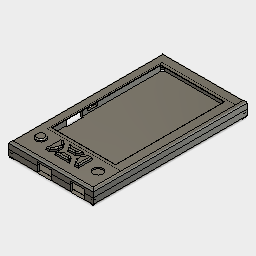
Case_Design (Autodesk Fusion 360 design; units mm, degrees)
Autodesk Fusion 360 part; units mm, degrees
sketch "Screen" plane through (0, 0, 0) normal (0, 1, 0) x (1, 0, 0)
  line L0 (-28.5, 49.35) -> (28.5, 49.35)
  line L1 (28.5, 49.35) -> (28.5, -49.35)
  line L2 (28.5, -49.35) -> (-28.5, -49.35)
  line L3 (-28.5, -49.35) -> (-28.5, 49.35)
  line L4 (-28.5, 49.35) -> (28.5, -49.35) construction
  line L5 (28.5, 49.35) -> (-28.5, -49.35) construction
  line L6 (-31.11, 52.75) -> (36.09, 52.75)
  line L7 (36.09, 52.75) -> (36.09, -52.75)
  line L8 (36.09, -52.75) -> (-31.11, -52.75)
  line L9 (-31.11, -52.75) -> (-31.11, 52.75)
  line L10 (29.5, 50.35) -> (-29.5, 50.35)
  line L11 (-29.5, 50.35) -> (-29.5, -50.35)
  line L12 (-29.5, -50.35) -> (29.5, -50.35)
  line L13 (29.5, -50.35) -> (29.5, 50.35)
  line L14 (29.5, 50.35) -> (-29.5, -50.35) construction
  line L15 (-29.5, 50.35) -> (29.5, -50.35) construction
  dimension "d1" = 98.7
  dimension "d2" = 57
  dimension "d3" = 31.11
  dimension "d4" = 36.09
  dimension "d5" = 52.75
  dimension "d6" = 52.75
  dimension "d14" = 100.7
  dimension "d15" = 59
  measures "d1" distance of L0.end L1.end
  measures "d2" distance of L1.end L2.end
  measures "d3" distance of origin L9
  measures "d4" distance of origin L7
  measures "d5" distance of origin L6
  measures "d6" distance of origin L8
  measures "d14" distance of L10.end L11.end
  measures "d15" distance of L11.end L12.end
extrude "Extrude1" add sketch "Screen" along normal blind 4.4 contours L6 L7 L8 L9 | L10 L11 L12 L13 picked at (33.893333, 16.783333) picked at (-29.166667, -16.45) makes body 1
extrude "Extrude2" add sketch "Screen" along normal blind 4.4 separate body contours L0 L1 L2 L3 picked at (-9.5, 16.45) makes body 2
extrude "Extrude3" add sketch "Screen" along normal blind 2 contours L0 L1 L2 L3 picked at (-9.5, 16.45) bodies 1
move_face "OffsetFaces1" offset -2 1 faces at (-9.5, 0, -16.45) on bodies 2
sketch "Board" plane through (0, 0, 0) normal (0, 1, 0) x (1, 0, 0)
  line L0 (-35.792, 11.9058) -> (36.09, 11.9058)
  line L1 (36.09, 11.9058) -> (36.09, -77.15)
  line L2 (36.09, -77.15) -> (-35.792, -77.15)
  line L3 (-35.792, -77.15) -> (-35.792, 11.9058)
  circle A0 centre (0.149, -59.1922) radius 2.25
  circle A1 centre (0.149, -68.0822) radius 2.25
  circle A2 centre (11.579, -63.6372) radius 2.25
  circle A3 centre (-11.281, -63.6372) radius 2.25
  circle A4 centre (-26.267, -63.6372) radius 2.25
  circle A5 centre (26.565, -63.6372) radius 2.25
  circle A6 centre (-31.651, -73.0942) radius 2
  circle A7 centre (31.949, -73.0942) radius 2
  line L4 (-35.792, -9.58404) -> (-32.192, -9.58404)
  line L5 (-32.192, -9.58404) -> (-32.192, -1.08404)
  line L6 (-32.192, -1.08404) -> (-35.792, -1.08404)
  line L7 (-35.792, -1.08404) -> (-35.792, -9.58404)
  line L8 (-35.792, -9.58404) -> (-32.192, -1.08404) construction
  line L9 (-32.192, -9.58404) -> (-35.792, -1.08404) construction
  line L10 (-35.792, -27.76274) -> (-23.292, -27.76274)
  line L11 (-23.292, -27.76274) -> (-23.292, -16.76274)
  line L12 (-23.292, -16.76274) -> (-35.792, -16.76274)
  line L13 (-35.792, -16.76274) -> (-35.792, -27.76274)
  line L14 (-35.792, -27.76274) -> (-23.292, -16.76274) construction
  line L15 (-23.292, -27.76274) -> (-35.792, -16.76274) construction
  line L16 (28.029, -77.15) -> (20.529, -77.15)
  line L17 (20.529, -77.15) -> (20.529, -71.4)
  line L18 (20.529, -71.4) -> (28.029, -71.4)
  line L19 (28.029, -71.4) -> (28.029, -77.15)
  line L20 (28.029, -77.15) -> (20.529, -71.4) construction
  line L21 (20.529, -77.15) -> (28.029, -71.4) construction
  line L22 (-2.451, -77.15) -> (-9.951, -77.15)
  line L23 (-9.951, -77.15) -> (-9.951, -71.4)
  line L24 (-9.951, -71.4) -> (-2.451, -71.4)
  line L25 (-2.451, -71.4) -> (-2.451, -77.15)
  line L26 (-2.451, -77.15) -> (-9.951, -71.4) construction
  line L27 (-9.951, -77.15) -> (-2.451, -71.4) construction
  line L28 (36.09, -52.75) -> (-31.11, -52.75)
  line L29 (-37.692, -1.441077) -> (-32.192, -1.441077)
  line L30 (-32.192, -1.441077) -> (-32.192, -3.441077)
  line L31 (-32.192, -3.441077) -> (-37.692, -3.441077)
  line L32 (-37.692, -3.441077) -> (-37.692, -1.441077)
  line L33 (-38.692, -17.26274) -> (-23.292, -17.26274)
  line L34 (-23.292, -17.26274) -> (-23.292, -27.26274)
  line L35 (-23.292, -27.26274) -> (-38.692, -27.26274)
  line L36 (-38.692, -27.26274) -> (-38.692, -17.26274)
  line L37 (-35.792, -77.15) -> (36.09, -77.15)
  line L38 (36.09, -77.15) -> (36.09, -40.95)
  line L39 (36.09, -40.95) -> (-35.792, -40.95)
  line L40 (-35.792, -40.95) -> (-35.792, -77.15)
  line L41 (-35.792, -1.08404) -> (-42.092, -1.08404)
  line L42 (-42.092, -1.08404) -> (-42.092, -9.58404)
  line L43 (-42.092, -9.58404) -> (-35.792, -9.58404)
  line L44 (-35.792, -9.58404) -> (-35.792, -1.08404)
  line L45 (-35.792, -27.76274) -> (-35.792, -16.76274)
  line L46 (-9.951, -77.15) -> (-2.451, -77.15)
  line L47 (20.529, -77.15) -> (28.029, -77.15)
  line L48 (-35.792, -14.76274) -> (-42.092, -14.76274)
  line L49 (-42.092, -14.76274) -> (-42.092, -29.76274)
  line L50 (-42.092, -29.76274) -> (-35.792, -29.76274)
  line L51 (-35.792, -29.76274) -> (-35.792, -14.76274)
  line L52 (-12.701, -77.15) -> (0.299, -77.15)
  line L53 (0.299, -77.15) -> (0.299, -83.45)
  line L54 (0.299, -83.45) -> (-12.701, -83.45)
  line L55 (-12.701, -83.45) -> (-12.701, -77.15)
  line L56 (17.779, -77.15) -> (30.779, -77.15)
  line L57 (30.779, -77.15) -> (30.779, -83.45)
  line L58 (30.779, -83.45) -> (17.779, -83.45)
  line L59 (17.779, -83.45) -> (17.779, -77.15)
  point P0 (-33.992, -5.33404)
  point P1 (-29.542, -22.26274)
  point P2 (24.279, -74.275)
  point P3 (-6.201, -74.275)
  dimension "d16" = 71.882
  dimension "d17" = 89.0558
  dimension "d18" = 4.5
  dimension "d19" = 17.9578
  dimension "d20" = 35.941
  dimension "d21" = 4.5
  dimension "d22" = 35.941
  dimension "d23" = 9.0678
  dimension "d24" = 4.5
  dimension "d25" = 13.5128
  dimension "d26" = 4.5
  dimension "d27" = 13.5128
  dimension "d28" = 4.5
  dimension "d29" = 13.5128
  dimension "d30" = 4.5
  dimension "d31" = 13.5128
  dimension "d32" = 11.43
  dimension "d33" = 11.43
  dimension "d34" = 26.416
  dimension "d35" = 26.416
  dimension "d36" = 4
  dimension "d37" = 4.141
  dimension "d38" = 4.0558
  dimension "d39" = 4
  dimension "d40" = 4.141
  dimension "d41" = 4.0558
  dimension "d42" = 17.23984
  dimension "d43" = 12.5
  dimension "d44" = 34.16854
  dimension "d45" = 7.5
  dimension "d46" = 5.75
  dimension "d47" = 11.811
  dimension "d48" = 5.75
  dimension "d49" = 7.5
  dimension "d50" = 5.75
  dimension "d51" = 5.75
  dimension "d52" = 42.291
  dimension "d53" = 36.09
  dimension "d54" = 24.4
  dimension "d57" = 11
  dimension "d58" = 8.5
  dimension "d59" = 3.6
  dimension "d60" = 5.5
  dimension "d61" = 2
  dimension "d62" = 5.5
  dimension "d63" = 15.4
  dimension "d64" = 10
  dimension "d65" = 15.4
  dimension "d66" = 0.5
  dimension "d80" = 36.2
  dimension "d129" = 6.3
  dimension "d161" = 6.3
  dimension "d162" = 15
  dimension "d164" = 2
  dimension "d177" = 13
  dimension "d178" = 6.3
  dimension "d179" = 13
  dimension "d180" = 6.3
  dimension "d181" = 2.75
  dimension "d182" = 2.75
  measures "d16" distance of L0.start L0.end
  measures "d17" distance of L0.start L2.end
  measures "d18" diameter of A0
  measures "d19" distance of L2 A0.centre
  measures "d20" distance of L1 A0.centre
  measures "d21" diameter of A1
  measures "d22" distance of L1 A1.centre
  measures "d23" distance of L2 A1.centre
  measures "d24" diameter of A2
  measures "d25" distance of L2 A2.centre
  measures "d26" diameter of A3
  measures "d27" distance of L2 A3.centre
  measures "d28" diameter of A4
  measures "d29" distance of L2 A4.centre
  measures "d30" diameter of A5
  measures "d31" distance of L2 A5.centre
  measures "d32" distance of A1.centre A3.centre
  measures "d33" distance of A1.centre A2.centre
  measures "d34" distance of A1.centre A4.centre
  measures "d35" distance of A1.centre A5.centre
  measures "d36" diameter of A6
  measures "d37" distance of L3 A6.centre
  measures "d38" distance of L2 A6.centre
  measures "d39" diameter of A7
  measures "d40" distance of L1 A7.centre
  measures "d41" distance of L2 A7.centre
  measures "d45" distance of L17.end L18.end
  measures "d46" distance of L16.end L17.end
  measures "d47" distance of L1 P2
  measures "d48" distance of L2 L18
  measures "d49" distance of L23.end L24.end
  measures "d50" distance of L22.end L23.end
  measures "d51" distance of L2 L24
  measures "d52" distance of L1 P3
  measures "d53" distance of origin L1
  measures "d54" distance of L2 L28
  measures "d57" distance of L10 L12
  measures "d58" distance of L4 L6
  measures "d59" distance of L3 L5
  measures "d62" distance of L5 L32
  measures "d65" distance of L11 L36
  measures "d66" distance of L12 L33
  measures "d80" distance of L2.end L39.end
  measures "d164" distance of L10 L50
  measures "d177" distance of L52.start L52.end
  measures "d178" distance of L52.start L54.end
  measures "d179" distance of L56.start L56.end
  measures "d180" distance of L56.start L58.end
  measures "d181" distance of L23 L55
  measures "d182" distance of L17 L59
extrude "Extrude4" add sketch "Board" against normal blind 1.65 separate body contours L0 L1 L3 L4 L5 L6 L10 L11 L12 L30 L34 L39 L51 | L3 L5 L6 L7 L29 L44 | L1 L2 L3 L17 L18 L19 L23 L24 L25 L37 L38 L39 L40 L52 L56 | L3 L5 L7 L29 L30 L31 L44 | L3 L4 L5 L7 L31 L44 | L3 L10 L11 L13 L35 L45 L51 | L2 L16 L17 L18 L19 L37 L47 L56 | L2 L22 L23 L24 L25 L37 L46 L52 | L3 L11 L13 L33 L34 L35 L45 L51 | L3 L11 L12 L13 L33 L45 L51 | A0 | A1 | A2 | A3 | A4 | A5 picked at (16.296, -15.26898) picked at (-33.392, -1.203052) picked at (0.092952, -46.28283) picked at (-33.392, -2.107744) picked at (-34.592, -7.536386) picked at (-27.458667, -27.596073) picked at (25.529, -73.316667) picked at (-4.951, -75.233333) picked at (-31.625333, -20.596073) picked at (-27.458667, -16.929407) picked at (0.092952, -58.767356) picked at (-0.017891, -67.351004) picked at (11.745891, -64.302315) picked at (-12.078671, -64.273321) picked at (-26.323048, -64.385103) picked at (26.621048, -64.351689) makes body 3
extrude "Extrude5" add sketch "Board" against normal blind 5.25 contours L3 L5 L6 L7 L29 L44 | L3 L5 L7 L29 L30 L31 L44 | L3 L7 L29 L31 L32 L44 | L3 L4 L5 L7 L31 L44 picked at (-33.392, -1.203052) picked at (-33.392, -2.107744) picked at (-37.058667, -2.774411) picked at (-34.592, -7.536386) bodies 3
extrude "Extrude6" add sketch "Board" against normal blind 3.1 contours L3 L10 L11 L13 L35 L45 L51 | L3 L13 L33 L35 L36 L45 L51 | L3 L11 L13 L33 L34 L35 L45 L51 | L3 L11 L12 L13 L33 L45 L51 picked at (-27.458667, -27.596073) picked at (-36.758667, -23.929407) picked at (-31.625333, -20.596073) picked at (-27.458667, -16.929407) bodies 3
extrude "Extrude7" cut sketch "Board" against normal blind 1.65 contours L3 L13 L33 L35 L36 L45 L51 picked at (-36.758667, -23.929407) bodies 3
extrude "Extrude8" cut sketch "Board" against normal blind 2.8 contours L3 L7 L29 L31 L32 L44 picked at (-37.058667, -2.774411) bodies 3
extrude "Extrude9" cut sketch "Board" along normal blind 0.45 from surface at -5.25 contours L3 L7 L29 L31 L32 L44 picked at (-37.058667, -2.774411) bodies 3
extrude "Extrude10" add sketch "Board" against normal blind 4.35 contours L2 L16 L17 L18 L19 L37 L47 L56 | L2 L22 L23 L24 L25 L37 L46 L52 picked at (25.529, -73.316667) picked at (-4.951, -75.233333) bodies 3
extrude "Extrude11" add sketch "Board" against normal blind 1.07 from surface at -5.15 separate body contours L1 L2 L3 L17 L18 L19 L23 L24 L25 L37 L38 L39 L40 L52 L56 | L2 L16 L17 L18 L19 L37 L47 L56 | L2 L22 L23 L24 L25 L37 L46 L52 | A0 | A1 | A2 | A3 | A4 | A5 | A6 picked at (0.092952, -46.28283) picked at (25.529, -73.316667) picked at (-4.951, -75.233333) picked at (0.092952, -58.767356) picked at (-0.017891, -67.351004) picked at (11.745891, -64.302315) picked at (-12.078671, -64.273321) picked at (-26.323048, -64.385103) picked at (26.621048, -64.351689) picked at (-31.140127, -73.843513) makes body 4
move_face "OffsetFaces2" offset 4 1 faces at (33.909345, -5.863333, 73.490492) on bodies 4
sketch "Case" plane through (0, 0, 0) normal (0, 1, 0) x (1, 0, 0)
  line L0 (-36.792, 59.65) -> (37.09, 59.65)
  line L1 (37.09, 59.65) -> (37.09, -78.65)
  line L2 (37.09, -78.65) -> (-36.792, -78.65)
  line L3 (-36.792, -78.65) -> (-36.792, 59.65)
  line L4 (36.09, 11.9058) -> (36.09, -77.15)
  line L5 (-35.792, -77.15) -> (36.09, -77.15)
  line L6 (-35.792, -40.95) -> (-35.792, -77.15)
  line L7 (-31.11, 52.75) -> (36.09, 52.75)
  line L8 (-38.792, 61.65) -> (39.09, 61.65)
  line L9 (39.09, 61.65) -> (39.09, -80.65)
  line L10 (39.09, -80.65) -> (-38.792, -80.65)
  line L11 (-38.792, -80.65) -> (-38.792, 61.65)
  circle A0 centre (-31.651, -73.0942) radius 1.35
  circle A1 centre (31.949, -73.0942) radius 1.35
  circle A2 centre (-31.651, -73.0942) radius 3
  circle A3 centre (31.949, -73.0942) radius 3
  circle A4 centre (-36.792, -78.65) radius 0.825
  circle A5 centre (-36.792, -78.65) radius 1.85
  circle A6 centre (37.09, -78.65) radius 0.825
  circle A7 centre (37.09, -78.65) radius 1.85
  circle A8 centre (-36.792, 59.65) radius 0.825
  circle A9 centre (-36.792, 59.65) radius 1.85
  circle A10 centre (37.09, 59.65) radius 0.825
  circle A11 centre (37.09, 59.65) radius 1.85
  line L12 (36.59, -77.65) -> (-36.292, -77.65)
  line L13 (-36.292, -77.65) -> (-36.292, -75.498152)
  line L14 (36.59, -77.65) -> (36.59, -75.817932)
  point P0 (-31.651, -73.0942)
  point P1 (31.949, -73.0942)
  dimension "d85" = 1
  dimension "d86" = 1.5
  dimension "d87" = 1
  dimension "d88" = 6.9
  dimension "d89" = 2
  dimension "d90" = 2
  dimension "d91" = 2
  dimension "d92" = 2
  dimension "d102" = 2.7
  dimension "d103" = 2.7
  dimension "d104" = 6
  dimension "d105" = 6
  dimension "d195" = 1.65
  dimension "d196" = 3.7
  dimension "d197" = 1.65
  dimension "d198" = 3.7
  dimension "d199" = 1.65
  dimension "d200" = 3.7
  dimension "d201" = 1.65
  dimension "d202" = 3.7
  dimension "d203" = 0.5
  dimension "d204" = 0.5
  dimension "d205" = 0.5
  measures "d85" distance of L1 L4
  measures "d86" distance of L2 L5
  measures "d87" distance of L3 L6
  measures "d88" distance of L0 L7
  measures "d89" distance of L2 L10
  measures "d90" distance of L1 L9
  measures "d91" distance of L3 L11
  measures "d92" distance of L0 L8
  measures "d102" diameter of A0
  measures "d103" diameter of A1
  measures "d104" diameter of A2
  measures "d105" diameter of A3
  measures "d195" diameter of A4
  measures "d196" diameter of A5
  measures "d197" diameter of A6
  measures "d198" diameter of A7
  measures "d199" diameter of A8
  measures "d200" diameter of A9
  measures "d201" diameter of A10
  measures "d202" diameter of A11
  measures "d203" distance of L6 L13
  measures "d204" distance of L5 L12
  measures "d205" distance of L4 L14
extrude "Extrude12" add sketch "Case" along normal blind 4.85 separate body contours L0 L3 A8 | L0 L3 A8 | L0 L3 A8 A9 | L0 L3 A8 A9 | L0 L1 L3 L5 A5 A7 A9 A11 | L0 L1 A10 A11 | L0 L1 A10 A11 | L2 L3 A4 A5 L12 L13 | L2 L3 A4 A5 | L0 L1 A10 | L0 L1 A10 | L2 L3 A4 | L2 L3 A4 | L5 L6 A5 L12 L13 | L2 A5 A7 L12 | L1 L2 A6 A7 | L1 L2 A6 A7 L12 L14 | L5 L6 A5 | L5 A5 A7 L12 | L1 L2 A6 | L1 L2 A6 | L4 L5 A7 L12 L14 | L4 L5 A7 | L8 L9 L10 L11 | A0 | A1 | A2 | A3 picked at (-37.189257, 59.27178) picked at (-36.244799, 59.610863) picked at (-38.236361, 60.070699) picked at (-35.906098, 58.433837) picked at (10.383659, 15.233899) picked at (35.591626, 59.782896) picked at (36.012293, 58.600037) picked at (-35.898689, -77.803247) picked at (-38.22667, -78.197355) picked at (36.852031, 60.144147) picked at (36.542799, 59.610863) picked at (-36.310506, -78.387085) picked at (-37.340345, -78.636539) picked at (-35.87162, -77.365492) picked at (11.846, -78.474515) picked at (35.588554, -78.741909) picked at (36.196689, -77.803247) picked at (-35.782685, -77.118479) picked at (11.943854, -77.526007) picked at (36.543072, -78.690987) picked at (36.575991, -78.458284) picked at (36.16962, -77.365492) picked at (36.080685, -77.118479) picked at (-37.006166, 12.933333) picked at (-31.751134, -72.655482) picked at (32.065167, -73.161269) picked at (-29.389022, -74.018087) picked at (29.687022, -74.018087) makes body 5
extrude "Extrude13" cut sketch "Screen" along normal blind 5 contours L0 L1 L2 L3 | L10 L11 L12 L13 picked at (-9.5, 16.45) picked at (-29.166667, -16.45) bodies 5
extrude "Extrude14" cut sketch "Screen" along normal blind 4.65 contours L0 L1 L2 L3 | L6 L7 L8 L9 | L10 L11 L12 L13 picked at (-9.5, 16.45) picked at (33.893333, 16.783333) picked at (-29.166667, -16.45) bodies 5
extrude "Extrude15" cut sketch "Case" along normal blind 4 contours L0 L3 A8 | L0 L3 A8 A9 | L0 L1 L3 L5 A5 A7 A9 A11 | L0 L1 A10 A11 | L2 L3 A4 A5 L12 L13 | L0 L1 A10 | L2 L3 A4 | L5 L6 A5 L12 L13 | L2 A5 A7 L12 | L1 L2 A6 A7 L12 L14 | L5 L6 A5 | L5 A5 A7 L12 | L1 L2 A6 | L4 L5 A7 L12 L14 | L4 L5 A7 | A0 | A1 | A2 | A3 picked at (-36.244799, 59.610863) picked at (-35.906098, 58.433837) picked at (10.383659, 15.233899) picked at (36.012293, 58.600037) picked at (-35.898689, -77.803247) picked at (36.542799, 59.610863) picked at (-36.310506, -78.387085) picked at (-35.87162, -77.365492) picked at (11.846, -78.474515) picked at (36.196689, -77.803247) picked at (-35.782685, -77.118479) picked at (11.943854, -77.526007) picked at (36.575991, -78.458284) picked at (36.16962, -77.365492) picked at (36.080685, -77.118479) picked at (-31.751134, -72.655482) picked at (32.065167, -73.161269) picked at (-29.389022, -74.018087) picked at (29.687022, -74.018087) bodies 5
extrude "Extrude16" add sketch "Case" along normal blind 4.45 contours A2 | A3 picked at (-29.389022, -74.018087) picked at (29.687022, -74.018087) bodies 5
move_face "OffsetFaces5" offset -1 1 faces at (36.09, 4.216667, -17.583333) on bodies 5
extrude "Extrude17" add 1 faces at (11.909948, 4, 58.851227) along direction (0, -1, 0) blind 0.2 on bodies 5 bodies 5
extrude "Extrude18" cut 1 faces at (14.356667, 4.366667, -52.75) along direction (0, 0, -1) blind 0.4 on bodies 5 bodies 5
extrude "Extrude19" add 1 faces at (9.932667, 4.85, 70.55) along direction (0, 1, 0) blind 0.2 on bodies 5 bodies 5
extrude "Extrude20" cut 2 faces at (32.029302, 4, 72.742376) (-31.550866, 4, 73.532918) along direction (0, 1, 0) blind 0.2 on bodies 5 bodies 5
extrude "Extrude21" cut 1 faces at (14.356667, 4.366667, -53.15) along direction (0, 0, -1) blind 0.05 on bodies 5 bodies 5
extrude "Extrude22" add 1 faces at (9.932667, 5.05, 70.55) along direction (0, 1, 0) blind 0.1 on bodies 5 bodies 5
extrude "Extrude23" cut 2 faces at (32.029302, 4.2, 72.742376) (-31.550866, 4.2, 73.532918) along direction (0, 1, 0) blind 0.1 on bodies 5 bodies 5
extrude "Extrude24" add sketch "Case" against normal blind 7.3 separate body contours L0 L3 A8 | L0 L3 A8 A9 | L0 L1 A10 A11 | L2 L3 A4 A5 | L0 L1 A10 | L2 L3 A4 | L1 L2 A6 A7 | L1 L2 A6 | L8 L9 L10 L11 picked at (-37.189257, 59.27178) picked at (-38.236361, 60.070699) picked at (35.591626, 59.782896) picked at (-38.22667, -78.197355) picked at (36.852031, 60.144147) picked at (-37.340345, -78.636539) picked at (35.588554, -78.741909) picked at (36.543072, -78.690987) picked at (-37.006166, 12.933333) makes body 6
extrude "Extrude25" add sketch "Case" against normal blind 0.5 from surface at -7.3 contours L0 L3 A8 | L0 L3 A8 | L0 L3 A8 A9 | L0 L3 A8 A9 | L0 L1 L3 L5 A5 A7 A9 A11 | L0 L1 A10 A11 | L0 L1 A10 A11 | L2 L3 A4 A5 L12 L13 | L2 L3 A4 A5 | L0 L1 A10 | L0 L1 A10 | L2 L3 A4 | L2 L3 A4 | L5 L6 A5 L12 L13 | L2 A5 A7 L12 | L1 L2 A6 A7 | L1 L2 A6 A7 L12 L14 | L5 L6 A5 | L5 A5 A7 L12 | L1 L2 A6 | L1 L2 A6 | L4 L5 A7 L12 L14 | L4 L5 A7 | L8 L9 L10 L11 | A0 | A1 | A2 | A3 picked at (-37.189257, 59.27178) picked at (-36.244799, 59.610863) picked at (-38.236361, 60.070699) picked at (-35.906098, 58.433837) picked at (10.383659, 15.233899) picked at (35.591626, 59.782896) picked at (36.012293, 58.600037) picked at (-35.898689, -77.803247) picked at (-38.22667, -78.197355) picked at (36.852031, 60.144147) picked at (36.542799, 59.610863) picked at (-36.310506, -78.387085) picked at (-37.340345, -78.636539) picked at (-35.87162, -77.365492) picked at (11.846, -78.474515) picked at (35.588554, -78.741909) picked at (36.196689, -77.803247) picked at (-35.782685, -77.118479) picked at (11.943854, -77.526007) picked at (36.543072, -78.690987) picked at (36.575991, -78.458284) picked at (36.16962, -77.365492) picked at (36.080685, -77.118479) picked at (-37.006166, 12.933333) picked at (-31.751134, -72.655482) picked at (32.065167, -73.161269) picked at (-29.389022, -74.018087) picked at (29.687022, -74.018087) bodies 6
extrude "Extrude26" cut sketch "Board" against normal blind 3 contours L0 L1 L3 L4 L5 L6 L10 L11 L12 L30 L34 L39 L51 | L3 L5 L6 L7 L29 L44 | L3 L7 L29 L31 L32 L41 L42 L43 L44 | L1 L2 L3 L17 L18 L19 L23 L24 L25 L37 L38 L39 L40 L52 L56 | L3 L5 L7 L29 L30 L31 L44 | L3 L7 L29 L31 L32 L44 | L3 L4 L5 L7 L31 L44 | L3 L10 L11 L13 L35 L45 L51 | L2 L16 L17 L18 L19 L37 L47 L56 | L2 L22 L23 L24 L25 L37 L46 L52 | L3 L11 L13 L33 L34 L35 L45 L51 | L3 L11 L12 L13 L33 L45 L51 | A0 | A1 | A2 | A3 | A4 | A5 | A6 | A7 picked at (16.296, -15.26898) picked at (-33.392, -1.203052) picked at (-38.525333, -7.536386) picked at (0.092952, -46.28283) picked at (-33.392, -2.107744) picked at (-37.058667, -2.774411) picked at (-34.592, -7.536386) picked at (-27.458667, -27.596073) picked at (25.529, -73.316667) picked at (-4.951, -75.233333) picked at (-31.625333, -20.596073) picked at (-27.458667, -16.929407) picked at (0.092952, -58.767356) picked at (-0.017891, -67.351004) picked at (11.745891, -64.302315) picked at (-12.078671, -64.273321) picked at (-26.323048, -64.385103) picked at (26.621048, -64.351689) picked at (-31.140127, -73.843513) picked at (32.579264, -73.579959) bodies 6
extrude "Extrude27" cut 2 faces at (-38.125333, -3, 3.917373) (-38.125333, -3, 3.917373) along direction (0, -1, 0) blind 2 on bodies 6 bodies 6
extrude "Extrude28" cut sketch "Board" against normal blind 3 contours L1 L2 L3 L17 L18 L19 L23 L24 L25 L37 L38 L39 L40 L52 L56 | L2 L16 L17 L18 L19 L37 L47 L56 | L2 L22 L23 L24 L25 L37 L46 L52 | A0 | A1 | A2 | A3 | A4 | A5 | A6 | A7 picked at (0.092952, -46.28283) picked at (25.529, -73.316667) picked at (-4.951, -75.233333) picked at (0.092952, -58.767356) picked at (-0.017891, -67.351004) picked at (11.745891, -64.302315) picked at (-12.078671, -64.273321) picked at (-26.323048, -64.385103) picked at (26.621048, -64.351689) picked at (-31.140127, -73.843513) picked at (32.579264, -73.579959) bodies 6
sketch "Buttons" plane through (0, 0, 0) normal (0, 1, 0) x (1, 0, 0)
  line L0 (3.649, -56.6922) -> (-3.351, -56.6922)
  line L1 (-3.351, -56.6922) -> (-3.351, -61.6922) construction
  line L2 (-3.351, -61.6922) -> (3.649, -61.6922)
  line L3 (3.649, -61.6922) -> (3.649, -56.6922) construction
  line L4 (3.649, -56.6922) -> (-3.351, -61.6922) construction
  line L5 (-3.351, -56.6922) -> (3.649, -61.6922) construction
  line L6 (3.649, -65.5822) -> (-3.351, -65.5822)
  line L7 (-3.351, -65.5822) -> (-3.351, -70.5822) construction
  line L8 (-3.351, -70.5822) -> (3.649, -70.5822)
  line L9 (3.649, -70.5822) -> (3.649, -65.5822) construction
  line L10 (3.649, -65.5822) -> (-3.351, -70.5822) construction
  line L11 (-3.351, -65.5822) -> (3.649, -70.5822) construction
  line L12 (3.649, -70.5822) -> (7.149, -70.5822)
  line L13 (-3.351, -70.5822) -> (-6.851, -70.5822)
  line L14 (-6.851, -70.5822) -> (-3.351, -65.5822)
  line L15 (7.149, -70.5822) -> (3.649, -65.5822)
  line L16 (3.649, -56.6922) -> (7.149, -56.6922)
  line L17 (-3.351, -56.6922) -> (-6.851, -56.6922)
  line L18 (-6.851, -56.6922) -> (-3.351, -61.6922)
  line L19 (7.149, -56.6922) -> (3.649, -61.6922)
  line L20 (15.079, -61.6872) -> (8.079, -61.6872) construction
  line L21 (8.079, -61.6872) -> (8.079, -65.5872)
  line L22 (8.079, -65.5872) -> (15.079, -65.5872) construction
  line L23 (15.079, -65.5872) -> (15.079, -61.6872)
  line L24 (15.079, -61.6872) -> (8.079, -65.5872) construction
  line L25 (8.079, -61.6872) -> (15.079, -65.5872) construction
  line L26 (8.079, -65.5872) -> (11.519774, -70.502592)
  line L27 (11.519774, -70.502592) -> (15.079, -70.502592)
  line L28 (8.079, -61.6872) -> (11.519774, -56.771808)
  line L29 (11.519774, -56.771808) -> (15.079, -56.771808)
  line L30 (15.079, -56.771808) -> (15.079, -61.6872)
  line L31 (15.079, -70.502592) -> (15.079, -65.5872)
  line L32 (-7.781, -61.6872) -> (-14.781, -61.6872) construction
  line L33 (-14.781, -61.6872) -> (-14.781, -65.5872)
  line L34 (-14.781, -65.5872) -> (-7.781, -65.5872) construction
  line L35 (-7.781, -65.5872) -> (-7.781, -61.6872)
  line L36 (-7.781, -61.6872) -> (-14.781, -65.5872) construction
  line L37 (-14.781, -61.6872) -> (-7.781, -65.5872) construction
  line L38 (-7.781, -61.6872) -> (-11.221774, -56.771808)
  line L39 (-11.221774, -56.771808) -> (-14.781, -56.771808)
  line L40 (-14.781, -56.771808) -> (-14.781, -61.6872)
  line L41 (-7.781, -65.5872) -> (-11.221774, -70.502592)
  line L42 (-11.221774, -70.502592) -> (-14.781, -70.502592)
  line L43 (-14.781, -70.502592) -> (-14.781, -65.5872)
  circle A0 centre (26.565, -63.6372) radius 4.5
  circle A1 centre (-26.267, -63.6372) radius 4.5
  circle A2 centre (-26.267, -63.6372) radius 4.3
  circle A3 centre (-26.267, -63.6372) radius 1.25
  circle A4 centre (-11.281, -63.6372) radius 1.25
  circle A5 centre (0.149, -59.1922) radius 1.25
  circle A6 centre (0.149, -68.0822) radius 1.25
  circle A7 centre (11.579, -63.6372) radius 1.25
  circle A8 centre (26.565, -63.6372) radius 4.3
  circle A9 centre (26.565, -63.6372) radius 1.25
  line L44 (-17.781, -53.6922) -> (18.079, -53.6922)
  line L45 (18.079, -53.6922) -> (18.079, -73.5822)
  line L46 (18.079, -73.5822) -> (-17.781, -73.5822)
  line L47 (-17.781, -73.5822) -> (-17.781, -53.6922)
  circle A10 centre (-26.267, -63.6372) radius 6.25
  line L48 (-5.759867, -57.0922) -> (5.562729, -57.0922)
  line L49 (-2.287861, -61.2922) -> (1.357745, -61.2922)
  line L50 (6.629845, -56.736333) -> (3.823255, -60.745747)
  line L51 (-6.297632, -56.785208) -> (-3.276985, -61.100418)
  line L52 (-2.287861, -61.2922) -> (-3.425784, -61.2922)
  line L53 (-3.276985, -61.100418) -> (-3.142738, -61.2922)
  line L54 (-5.759867, -57.0922) -> (-6.54032, -57.0922)
  line L55 (-6.297632, -56.785208) -> (-6.303023, -56.777508)
  line L56 (5.562729, -57.0922) -> (6.380738, -57.0922)
  line L57 (3.823255, -60.745747) -> (3.3493, -61.422826)
  line L58 (1.357745, -61.2922) -> (3.440738, -61.2922)
  line L59 (8.479, -62.046318) -> (8.479, -65.111551)
  line L60 (8.740137, -65.834164) -> (11.725664, -70.099203)
  line L61 (12.282208, -70.102592) -> (14.522186, -70.102592)
  line L62 (14.679, -69.606243) -> (14.679, -57.595836)
  line L63 (14.536922, -57.171808) -> (12.223261, -57.171808)
  line L64 (11.623844, -57.320655) -> (8.695281, -61.504316)
  line L65 (14.679, -57.595836) -> (14.679, -56.836265)
  line L66 (11.623844, -57.320655) -> (11.970044, -56.826083)
  line L67 (8.695281, -61.504316) -> (8.202168, -62.208763)
  line L68 (8.740137, -65.834164) -> (8.205868, -65.070923)
  line L69 (8.479, -65.111551) -> (8.479, -65.461111)
  line L70 (12.282208, -70.102592) -> (11.477234, -70.102592)
  line L71 (11.725664, -70.099203) -> (11.728036, -70.102592)
  line L72 (14.679, -69.606243) -> (14.679, -70.426864)
  line L73 (14.522186, -70.102592) -> (14.679, -70.102592)
  line L74 (14.536922, -57.171808) -> (14.679, -57.171808)
  line L75 (12.223261, -57.171808) -> (11.728036, -57.171808)
  line L76 (-6.405298, -70.643) -> (-3.068324, -65.875894)
  line L77 (-2.80703, -65.9822) -> (3.520319, -65.9822)
  line L78 (3.628301, -66.250147) -> (6.683218, -70.614314)
  line L79 (6.421738, -70.1822) -> (-5.596015, -70.1822)
  line L80 (-5.596015, -70.1822) -> (-6.082738, -70.1822)
  line L81 (-2.80703, -65.9822) -> (-3.142738, -65.9822)
  line L82 (3.520319, -65.9822) -> (3.713792, -65.9822)
  line L83 (3.628301, -66.250147) -> (3.440738, -65.9822)
  line L84 (6.421738, -70.1822) -> (6.380738, -70.1822)
  line L85 (-14.381, -56.925456) -> (-14.381, -70.342445)
  line L86 (-14.262215, -70.102592) -> (-11.314217, -70.102592)
  line L87 (-11.291819, -69.905138) -> (-8.288132, -65.614157)
  line L88 (-8.181, -62.073669) -> (-8.181, -65.194233)
  line L89 (-8.293888, -61.652021) -> (-11.525249, -57.03579)
  line L90 (-11.515543, -57.171808) -> (-14.391639, -57.171808)
  line L91 (-14.391639, -57.171808) -> (-14.381, -57.171808)
  line L92 (-11.515543, -57.171808) -> (-11.430036, -57.171808)
  line L93 (-8.181, -62.073669) -> (-8.181, -61.516626)
  line L94 (-8.293888, -61.652021) -> (-8.181, -61.813289)
  line L95 (-8.181, -65.194233) -> (-8.181, -65.701633)
  line L96 (-8.288132, -65.614157) -> (-8.181, -65.461111)
  line L97 (-11.314217, -70.102592) -> (-11.175918, -70.102592)
  line L98 (-11.291819, -69.905138) -> (-11.430036, -70.102592)
  line L99 (-14.262215, -70.102592) -> (-14.381, -70.102592)
  line L100 (8.479, -62.046318) -> (8.479, -61.813289)
  point P0 (0.149, -59.1922)
  point P1 (0.149, -59.1922)
  point P2 (0.149, -68.0822)
  point P3 (0.149, -68.0822)
  point P4 (11.579, -63.6372)
  point P5 (11.579, -63.6372)
  point P6 (-11.281, -63.6372)
  point P7 (-11.281, -63.6372)
  point P8 (26.565, -63.6372)
  point P9 (-26.267, -63.6372)
  dimension "d143" = 5
  dimension "d144" = 7
  dimension "d145" = 5
  dimension "d146" = 7
  dimension "d147" = 3.5
  dimension "d148" = 3.5
  dimension "d149" = 3.5
  dimension "d150" = 3.5
  dimension "d151" = 3.9
  dimension "d152" = 7
  dimension "d153" = 6
  dimension "d154" = 6
  dimension "d155" = 7
  dimension "d156" = 3.9
  dimension "d157" = 6
  dimension "d158" = 6
  dimension "d159" = 9
  dimension "d160" = 9
  dimension "d252" = 8.6
  dimension "d256" = 2.5
  dimension "d257" = 2.5
  dimension "d258" = 2.5
  dimension "d259" = 2.5
  dimension "d260" = 2.5
  dimension "d261" = 8.6
  dimension "d262" = 2.5
  dimension "d263" = 3
  dimension "d264" = 3
  dimension "d265" = 3
  dimension "d266" = 3
  dimension "d267" = 12.5
  dimension "d278" = 0.4
  dimension "d279" = 0.4
  dimension "d280" = 0.4
  dimension "d281" = 0.4
  dimension "d282" = 0.4
  dimension "d283" = 0.4
  dimension "d284" = 0.4
  dimension "d285" = 0.4
  dimension "d286" = 0.4
  dimension "d287" = 0.4
  dimension "d288" = 0.4
  dimension "d289" = 0.4
  dimension "d290" = 0.4
  dimension "d291" = 0.4
  dimension "d292" = 0.4
  dimension "d293" = 0.4
  dimension "d294" = 0.4
  dimension "d295" = 0.4
  dimension "d296" = 0.4
  dimension "d297" = 0.4
  measures "d143" distance of L0.end L1.end
  measures "d144" distance of L1.end L2.end
  measures "d145" distance of L6.end L7.end
  measures "d146" distance of L7.end L8.end
  measures "d147" distance of L8.end L12.end
  measures "d148" distance of L7.end L13.end
  measures "d149" distance of L0.start L16.end
  measures "d150" distance of L0.end L17.end
  measures "d151" distance of L20.end L21.end
  measures "d152" distance of L21.end L22.end
  measures "d155" distance of L33.end L34.end
  measures "d156" distance of L32.end L33.end
  measures "d159" diameter of A0
  measures "d160" diameter of A1
  measures "d252" diameter of A2
  measures "d256" diameter of A3
  measures "d257" diameter of A4
  measures "d258" diameter of A5
  measures "d259" diameter of A6
  measures "d260" diameter of A7
  measures "d261" diameter of A8
  measures "d262" diameter of A9
  measures "d263" distance of L0 L44
  measures "d264" distance of L8 L46
  measures "d265" distance of L23 L45
  measures "d266" distance of L33 L47
  measures "d267" diameter of A10
  measures "d278" distance of L0 L48
  measures "d279" distance of L2 L49
  measures "d280" distance of L19 L50
  measures "d281" distance of L18 L51
  measures "d282" distance of L28 L64
  measures "d283" distance of L29 L63
  measures "d284" distance of L30 L62
  measures "d285" distance of L27 L61
  measures "d286" distance of L26 L60
  measures "d287" distance of L21 L59
  measures "d288" distance of L14 L76
  measures "d289" distance of L6 L77
  measures "d290" distance of L15 L78
  measures "d291" distance of L13 L79
  measures "d292" distance of L43 L85
  measures "d293" distance of L42 L86
  measures "d294" distance of L41 L87
  measures "d295" distance of L35 L88
  measures "d296" distance of L38 L89
  measures "d297" distance of L39 L90
extrude "Extrude30" cut sketch "Buttons" along normal blind 6 contours L0 L2 L16 L17 L18 L19 | L6 L12 L13 L14 L15 L76 L77 L78 L81 L83 | L8 L12 L13 L76 L78 L79 L80 | L76 L77 L78 L79 L80 L81 L83 | L21 L23 L26 L27 L28 L29 L30 L31 | L33 L35 L38 L39 L40 L41 L42 L43 | A0 | A1 | A2 | A3 | A4 | A5 | A6 | A7 | A8 | A9 | L48 L49 L50 L51 L52 L53 L54 L56 L57 L58 | L59 L60 L61 L62 L63 L64 L65 L66 L67 L68 L69 L70 L71 L72 L73 L74 L75 L100 | L85 L86 L87 L88 L89 L90 L92 L93 L94 L95 L96 L98 L99 picked at (-1.182713, -56.958867) picked at (5.726246, -68.7822) picked at (-0.855426, -70.315533) picked at (-3.275264, -68.144301) picked at (14.812333, -64.263093) picked at (-14.514333, -62.9872) picked at (25.36426, -67.893299) picked at (-23.338519, -66.950831) picked at (-23.00433, -63.912928) picked at (-26.007213, -63.78087) picked at (-11.373717, -63.321732) picked at (-0.516997, -59.502625) picked at (0.117862, -68.967135) picked at (11.838787, -63.78087) picked at (29.82767, -63.912928) picked at (26.824787, -63.78087) picked at (-3.37463, -59.066172) picked at (10.588883, -66.929742) picked at (-12.43057, -68.269507) bodies 5
extrude "Extrude31" add 1 faces at (38.423333, 0, 32.55) along direction (0, -1, 0) blind 1.67 on bodies 5 bodies 5
extrude "Extrude32" cut sketch "Board" along normal blind 0.5 from surface at -1.67 contours L3 L13 L33 L35 L36 L45 L48 L49 L50 L51 | L3 L13 L33 L35 L36 L45 L51 picked at (-40.958667, -23.929407) picked at (-36.758667, -23.929407) bodies 5
extrude "Extrude33" cut 3 faces at (38.423333, 0, 32.55) (38.423333, 0, 32.55) (38.423333, 0, 32.55) along direction (0, -1, 0) blind 1.67 on bodies 6 bodies 6
extrude "Extrude34" cut sketch "Board" against normal blind 8 contours L3 L13 L33 L35 L36 L45 L48 L49 L50 L51 | L3 L13 L33 L35 L36 L45 L51 picked at (-40.958667, -23.929407) picked at (-36.758667, -23.929407) bodies 6
fillet "Fillet1" radius 2 5 edges at (0.149, -7.8, -61.65) (39.09, -7.8, 9.5) (0.149, -7.8, 80.65) (-38.792, -7.8, 55.20637) (-38.792, -7.8, -23.44363) on bodies 6
extrude "Extrude35" cut sketch "Board" against normal blind 3 from surface at -4.35 contours L2 L22 L37 L46 L52 L53 L54 L55 picked at (-4.951, -81.35) bodies 6
extrude "Extrude36" cut sketch "Board" against normal blind 3 from surface at -4.35 contours L2 L16 L37 L47 L56 L57 L58 L59 picked at (25.529, -81.35) bodies 6
extrude "Extrude37" cut sketch "Board" along normal blind 3 from surface at -1.65 contours L2 L16 L37 L47 L56 L57 L58 L59 | L2 L22 L37 L46 L52 L53 L54 L55 picked at (25.529, -81.35) picked at (-4.951, -81.35) bodies 5
extrude "Extrude38" cut 2 faces at (-8.367667, -4.35, 79.983333) (22.112333, -4.35, 79.316667) along direction (0, 1, 0) blind 3 on bodies 6 bodies 5 6
fillet "Fillet2" radius 2 4 edges at (-38.792, 5.15, 9.5) (0.149, 5.15, 80.65) (39.09, 5.15, 9.5) (0.149, 5.15, -61.65) on bodies 5
extrude "Extrude39" add sketch "Case" against normal blind 5.5 from surface at 3.8 contours L1 L2 A6 A7 | L1 L2 A6 A7 L12 L14 picked at (35.588554, -78.741909) picked at (36.196689, -77.803247) bodies 5
extrude "Extrude40" cut 1 faces at (36.202931, -1.7, 77.796286) along direction (0, 1, 0) blind 0.03 on bodies 5 bodies 5
extrude "Extrude41" cut sketch "Case" against normal blind 6.6 from surface at 3.8 contours L1 L2 A6 | L1 L2 A6 picked at (36.543072, -78.690987) picked at (36.575991, -78.458284) bodies 5
extrude "Extrude42" add sketch "Case" against normal blind 5.47 from surface at 3.8 contours L2 L3 A4 A5 L12 L13 | L2 L3 A4 A5 picked at (-35.898689, -77.803247) picked at (-38.22667, -78.197355) bodies 5
extrude "Extrude43" cut sketch "Case" against normal blind 7 from surface at 3.8 contours L2 L3 A4 | L2 L3 A4 picked at (-36.310506, -78.387085) picked at (-37.340345, -78.636539) bodies 5
extrude "Extrude44" add sketch "Case" against normal blind 5.47 from surface at 3.8 contours L0 L3 A8 A9 | L0 L3 A8 A9 picked at (-38.236361, 60.070699) picked at (-35.906098, 58.433837) bodies 5
extrude "Extrude45" cut sketch "Case" against normal blind 9 from surface at 3.8 contours L0 L3 A8 | L0 L3 A8 picked at (-37.189257, 59.27178) picked at (-36.244799, 59.610863) bodies 5
extrude "Extrude46" add sketch "Case" against normal blind 5.47 from surface at 3.8 contours L0 L1 A10 A11 | L0 L1 A10 A11 picked at (35.591626, 59.782896) picked at (36.012293, 58.600037) bodies 5
extrude "Extrude47" cut sketch "Case" against normal blind 8.2 from surface at 3.8 contours L0 L1 A10 | L0 L1 A10 picked at (36.852031, 60.144147) picked at (36.542799, 59.610863) bodies 5
delete_face "DeleteFace1" 5 faces at (-37.013976, -7.787643, 62.48071) (-37.013976, -7.787643, -34.972217) (12.462667, -7.783833, 78.903783) (38.437597, -7.277831, 32.922351) (-12.164667, -7.783833, -59.903783) on bodies 6
extrude "Extrude48" add 1 faces at (14.129333, -7.8, 11.254247) along direction (0, -1, 0) blind 1 on bodies 6 bodies 6
fillet "Fillet3" radius 2 5 edges at (-38.792, -8.8, 55.20637) (0.149, -8.8, 80.65) (39.09, -8.8, 9.5) (0.149, -8.8, -61.65) (-38.792, -8.8, -23.44363) on bodies 6
extrude "Extrude49" add sketch "Case" along normal blind 5.63 from surface at -7.3 contours L0 L3 A8 A9 | L0 L3 A8 A9 | L0 L1 A10 A11 | L0 L1 A10 A11 | L2 L3 A4 A5 L12 L13 | L2 L3 A4 A5 | L1 L2 A6 A7 | L1 L2 A6 A7 L12 L14 picked at (-38.236361, 60.070699) picked at (-35.906098, 58.433837) picked at (35.591626, 59.782896) picked at (36.012293, 58.600037) picked at (-35.898689, -77.803247) picked at (-38.22667, -78.197355) picked at (35.588554, -78.741909) picked at (36.196689, -77.803247) bodies 6
extrude "Extrude50" cut sketch "Case" along normal blind 11 from surface at -7.3 contours L0 L3 A8 | L0 L3 A8 | L0 L1 A10 | L0 L1 A10 | L2 L3 A4 | L1 L2 A6 picked at (-37.189257, 59.27178) picked at (-36.244799, 59.610863) picked at (36.852031, 60.144147) picked at (36.542799, 59.610863) picked at (-37.340345, -78.636539) picked at (36.543072, -78.690987) bodies 6
extrude "Extrude51" cut 1 faces at (-38.125333, -5, 3.917373) along direction (0, -1, 0) blind 0.5 on bodies 6 bodies 6
extrude "Extrude52" cut sketch "Case" along normal blind 5.03 from surface at -8.8 contours L0 L3 A8 | L0 L3 A8 | L0 L3 A8 A9 | L0 L3 A8 A9 | L0 L1 A10 A11 | L0 L1 A10 A11 | L2 L3 A4 A5 L12 L13 | L2 L3 A4 A5 | L0 L1 A10 | L0 L1 A10 | L2 L3 A4 | L2 L3 A4 | L5 L6 A5 L12 L13 | L1 L2 A6 A7 | L1 L2 A6 A7 L12 L14 | L1 L2 A6 | L1 L2 A6 | L4 L5 A7 L12 L14 picked at (-37.189257, 59.27178) picked at (-36.244799, 59.610863) picked at (-38.236361, 60.070699) picked at (-35.906098, 58.433837) picked at (35.591626, 59.782896) picked at (36.012293, 58.600037) picked at (-35.898689, -77.803247) picked at (-38.22667, -78.197355) picked at (36.852031, 60.144147) picked at (36.542799, 59.610863) picked at (-36.310506, -78.387085) picked at (-37.340345, -78.636539) picked at (-35.87162, -77.365492) picked at (35.588554, -78.741909) picked at (36.196689, -77.803247) picked at (36.543072, -78.690987) picked at (36.575991, -78.458284) picked at (36.16962, -77.365492) bodies 6
extrude "Extrude53" cut sketch "Case" against normal blind 10 from surface at -7.3 contours L5 L6 A5 picked at (-35.782685, -77.118479) bodies 6
extrude "Extrude54" cut sketch "Case" against normal blind 10 from surface at -7.3 contours L4 L5 A7 picked at (36.080685, -77.118479) bodies 6
extrude "Extrude55" add sketch "Buttons" along normal blind 7.5 from surface at 0.55 separate body contours A2 | A3 picked at (-23.00433, -63.912928) picked at (-26.007213, -63.78087) makes body 7
extrude "Extrude56" add sketch "Buttons" along normal blind 2.5 from surface at 0.55 contours A1 | A2 | A3 | A10 picked at (-23.338519, -66.950831) picked at (-23.00433, -63.912928) picked at (-26.007213, -63.78087) picked at (-20.640356, -64.171268) bodies 7
extrude "Extrude57" cut sketch "Buttons" along normal blind 1.5 contours A1 | A2 | A10 picked at (-23.338519, -66.950831) picked at (-23.00433, -63.912928) picked at (-20.640356, -64.171268) bodies 7
extrude "Extrude58" add 1 faces at (-26.162205, 0.55, 63.926574) along direction (0, -1, 0) blind 1 on bodies 7 bodies 7
extrude "Extrude59" cut 1 faces at (-26.585947, 8.05, 62.366092) along direction (0, -1, 0) blind 1 on bodies 7 bodies 7
fillet "Fillet4" radius 1 1 edges at (-30.276008, 7.05, 62.082254) on bodies 7
extrude "Extrude60" add sketch "Buttons" along normal blind 7.5 separate body contours L0 L2 L16 L17 L18 L19 | L6 L12 L13 L14 L15 L76 L77 L78 L81 L83 | L8 L12 L13 L76 L78 L79 L80 | L76 L77 L78 L79 L80 L81 L83 | L21 L23 L26 L27 L28 L29 L30 L31 | L33 L35 L38 L39 L40 L41 L42 L43 | A4 | A5 | A6 | A7 | L44 L45 L46 L47 | L48 L49 L50 L51 L52 L53 L54 L56 L57 L58 | L59 L60 L61 L62 L63 L64 L65 L66 L67 L68 L69 L70 L71 L72 L73 L74 L75 L100 | L85 L86 L87 L88 L89 L90 L92 L93 L94 L95 L96 L98 L99 picked at (-1.182713, -56.958867) picked at (5.726246, -68.7822) picked at (-0.855426, -70.315533) picked at (-3.275264, -68.144301) picked at (14.812333, -64.263093) picked at (-14.514333, -62.9872) picked at (-11.373717, -63.321732) picked at (-0.516997, -59.502625) picked at (0.117862, -68.967135) picked at (11.838787, -63.78087) picked at (1.315667, -72.5822) picked at (-3.37463, -59.066172) picked at (10.588883, -66.929742) picked at (-12.43057, -68.269507) makes body 8
extrude "Extrude61" cut sketch "Buttons" along normal blind 1.95 contours L0 L2 L16 L17 L18 L19 | L6 L12 L13 L14 L15 L76 L77 L78 L81 L83 | L8 L12 L13 L76 L78 L79 L80 | L76 L77 L78 L79 L80 L81 L83 | L21 L23 L26 L27 L28 L29 L30 L31 | L33 L35 L38 L39 L40 L41 L42 L43 | L44 L45 L46 L47 | L48 L49 L50 L51 L52 L53 L54 L56 L57 L58 | L59 L60 L61 L62 L63 L64 L65 L66 L67 L68 L69 L70 L71 L72 L73 L74 L75 L100 | L85 L86 L87 L88 L89 L90 L92 L93 L94 L95 L96 L98 L99 picked at (-1.182713, -56.958867) picked at (5.726246, -68.7822) picked at (-0.855426, -70.315533) picked at (-3.275264, -68.144301) picked at (14.812333, -64.263093) picked at (-14.514333, -62.9872) picked at (1.315667, -72.5822) picked at (-3.37463, -59.066172) picked at (10.588883, -66.929742) picked at (-12.43057, -68.269507) bodies 8
extrude "Extrude62" cut sketch "Buttons" against normal blind 4 from surface at 7.5 contours L0 L2 L16 L17 L18 L19 | L6 L12 L13 L14 L15 L76 L77 L78 L81 L83 | L8 L12 L13 L76 L78 L79 L80 | L21 L23 L26 L27 L28 L29 L30 L31 | L33 L35 L38 L39 L40 L41 L42 L43 | L44 L45 L46 L47 picked at (-1.182713, -56.958867) picked at (5.726246, -68.7822) picked at (-0.855426, -70.315533) picked at (14.812333, -64.263093) picked at (-14.514333, -62.9872) picked at (1.315667, -72.5822) bodies 8
fillet "Fillet5" radius 1 20 edges at (0.149, 7.5, 57.0922) (-4.612738, 7.5, 59.1922) (0.149, 7.5, 61.2922) (4.910738, 7.5, 59.1922) (13.203518, 7.5, 57.171808) (10.103518, 7.5, 59.492549) (8.479, 7.5, 63.6372) (10.103518, 7.5, 67.781851) (13.203518, 7.5, 70.102592) (14.679, 7.5, 63.6372) (0.149, 7.5, 70.1822) (-4.612738, 7.5, 68.0822) (0.149, 7.5, 65.9822) (4.910738, 7.5, 68.0822) (-9.805518, 7.5, 59.492549) (-12.905518, 7.5, 57.171808) (-14.381, 7.5, 63.6372) (-9.805518, 7.5, 67.781851) (-8.181, 7.5, 63.6372) (-12.905518, 7.5, 70.102592) on bodies 8
extrude "Extrude63" cut 4 faces at (-11.373717, 0, 63.321732) (0.117862, 0, 68.967135) (-0.516997, 0, 59.502625) (11.838787, 0, 63.78087) along direction (0, 1, 0) blind 0.4 on bodies 8 bodies 8
hidden bodies 1 2 3 4
equation "d5 = ( 105.5 / 2 ) * 1 mm"
equation "d6 = ( 105.5 / 2 ) * 1 mm"
equation "d73 = -4.8 mm + 2 mm"
equation "d81 = -3.50 mm - 1.65 mm"
equation "d88 = 1 mm + 5.9 mm"
equation "d215 = -5.50 mm + 0.03 mm"
equation "d221 = -5.50 mm + 0.03 mm"
equation "d227 = -5.50 mm + 0.03 mm"
equation "d298 = 1.95 mm + 1.55 mm + 4 mm"
named bodies: "Screen Casing", "Screen", "Board", "CM3L", "Case Front", "Case Back", "Button B", "Button Arrows"
